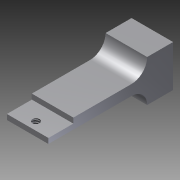
# Autodesk Inventor part: headplateHolder
Saved by Autodesk Inventor 2012 (Build 160160000, 160)
## iProperties
Created: 2011-10-06
Part Number: headplateHolder
Material: Default
Document SubType Name: Modeling
Designer: charvey
Density: 1 g/cm^3
Author: charvey
Autodesk Inventor part; units mm, degrees
ref_plane "YZ Plane" through (0, 0, 0) normal (1, 0, 0) x (0, 1, 0)
ref_plane "XZ Plane" through (0, 0, 0) normal (0, 1, 0) x (-1, 0, 0)
sketch "Sketch1" plane through (0, 0, 0) normal (0, 0, 1) x (1, 0, 0)
  line L0 (-6.35, 6.35) -> (6.35, 6.35)
  line L1 (6.35, 6.35) -> (6.35, -6.35)
  line L2 (6.35, -6.35) -> (-6.35, -6.35)
  line L3 (-6.35, -6.35) -> (-6.35, 6.35)
  point P0 (0, 0)
  point P1 (0, 6.35)
  point P2 (-6.35, 0)
  dimension "d0" = 12.7
  dimension "d1" = 12.7
  constraints: 8 end point, 2 midpoint, 2 parallel, 1 horizontal, 1 horizontal alignment, 1 perpendicular, 1 vertical alignment
  measures "d0" distance between parallel lines of L1 L3
  measures "d1" distance between parallel lines of L2 L0
extrude "Extrusion1" add sketch "Sketch1" along normal blind 38.1
ref_plane "Work Plane1" through (19.05, -6.35, 0) normal (1, 0, 0) x (0, 0, -1)
sketch "Sketch2" plane through (19.05, -6.35, 0) normal (1, 0, 0) x (0, 0, -1)
  line L0 (-38.1, 12.7) -> (-38.1, 0) projected
  line L1 (0, 0) -> (-38.1, 0) projected
  line L2 (0, 12.7) -> (0, 0) projected
  line L3 (0, 12.7) -> (-38.1, 12.7) projected
  line L4 (-38.1, 7.9375) -> (-12.7, 7.9375)
  arc A0 (-12.7, 7.9375) -> (-7.9375, 12.7) centre (-12.7, 12.7) ccw
  point P0 (0, 6.35)
  dimension "d5" = 25.4
  dimension "d6" = 1.5875
  dimension "d7" = 4.7625
  constraints: 2 end point, 2 point on circle, 2 point on line, 1 centre point, 1 parallel, 1 vertical alignment
  measures "d5" distance of L4.end L4.start
  measures "d6" distance from line of point (0, 6.35) L4
  measures "d7" radius of A0
extrude "Extrusion2" cut sketch "Sketch2" against normal blind 38.1 contours L3 A0 L4 L0
mirror "Mirror1" about plane through (0, 0, 0) normal (0, 1, 0) of "Extrusion2"
sketch "Sketch3" plane through (19.05, -6.35, 0) normal (1, 0, 0) x (0, 0, -1)
  arc A0 (-7.9375, 0) -> (-12.7, 4.7625) centre (-12.7, 0) ccw projected
  line L0 (0, 0) -> (-7.9375, 0) projected
  line L1 (0, 12.7) -> (0, 0) projected
  line L2 (0, 12.7) -> (-7.9375, 12.7) projected
  arc A1 (-12.7, 7.9375) -> (-7.9375, 12.7) centre (-12.7, 12.7) ccw projected
  line L3 (-12.7, 7.9375) -> (-38.1, 7.9375) projected
  line L4 (-38.1, 7.9375) -> (-38.1, 4.7625) projected
  line L5 (-38.1, 4.7625) -> (-12.7, 4.7625) projected
  line L6 (-30.48, 7.9375) -> (-30.48, 6.35)
  line L7 (-30.48, 6.35) -> (-38.1, 6.35)
  point P0 (0, 6.35)
  dimension "d10" = 1.5875
  dimension "d11" = 7.62
  constraints: 4 end point, 1 midpoint, 1 perpendicular, 1 point on line
  measures "d10" distance of L6.end L6.start
  measures "d11" distance between parallel lines of L6 L4
extrude "Extrusion3" cut sketch "Sketch3" against normal blind 38.1 contours L4 L3 L6 L7
sketch "Sketch4" plane through (-6.35, 0, 30.48) normal (0, 1, 0) x (1, 0, 0)
  line L0 (0, -7.62) -> (0, 0) projected
  line L1 (12.7, -7.62) -> (0, -7.62) projected
  point P0 (6.35, 30.48)
  point P1 (6.35, -5.08)
  dimension "d14" = 6.35
  dimension "d15" = 2.54
  measures "d14" distance from line of L0 point (6.35, -5.08)
  measures "d15" distance from line of L1 point (6.35, -5.08)
hole "Hole1" at (0, 0, 35.56) direction (0, -1, 0) diameter 2.159 end through all
sketch "Sketch5" plane through (0, 0, 0) normal (0, 0, -1) x (-1, 0, 0)
  point P0 (0, 0)
  point P1 (0, 0)
  constraints: 1 coincident
hole "Hole2" at (0, 0, 0) direction (0, 0, 1) diameter 3.302 depth 7.62 tip angle 118 thread size "8-32 UNC" class "2B" standard "ANSI Unified Screw Threads"
body "Solid1"
